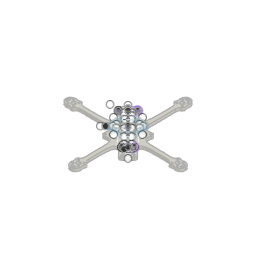
grognatiny (Autodesk Fusion 360 design; units mm, degrees)
Autodesk Fusion 360 part; units mm, degrees
(part 1 of 2)
sketch "Sketch1" plane through (0, 0, 0) normal (0, 0, 1) x (1, 0, 0)
  circle A0 centre (55.82676, 0) radius 4.5 construction
  line L0 (0, 0) -> (55.82676, 0) construction
  line L1 (55.82676, 0) -> (52.64478, 3.181981) construction
  line L2 (219.66262, 222.035886) -> (219.66262, 222.035886)
  circle A1 centre (52.64478, 3.181981) radius 1.05
  circle A2 centre (55.82676, 0) radius 2.25
  line L3 (45.82676, 2) -> (45.82676, -2) construction
  line L4 (55.82676, 0) -> (61.381639, 0) construction
  spline S0 degree 5 poles (60.950506, 0) (60.950506, -0.153969) (60.950156, -0.460974) (60.948561, -0.918704) (60.952621, -1.510726) (61.007799, -2.153667) (61.155369, -2.62162) (61.412622, -2.857725) (61.767904, -2.839751) (62.117367, -2.642136) (62.39542, -2.343591) (62.593133, -1.996472) (62.724237, -1.640351) (62.815846, -1.297091) (62.886296, -0.972425) (62.940492, -0.658247) (62.96936, -0.404167) (62.980649, -0.205879) (62.983159, -0.06935) (62.983159, 0) knots 0 0 0 0 0 0 0.06666667 0.13333333 0.2 0.26666667 0.33333333 0.4 0.46666667 0.53333333 0.6 0.66666667 0.73333333 0.8 0.86666667 0.93333333 1 1 1 1 1 1
  line L5 (60.950506, 0.838643) -> (60.950506, -0.838643)
  line L6 (62.983159, -0.583098) -> (62.983159, 0.583098)
  line L7 (61.359965, -2.867913) -> (62.011175, -2.759378)
  spline S1 degree 5 poles (64.574603, 0) (64.572644, 0.038801) (64.562798, 0.142773) (64.530239, 0.377838) (64.452884, 0.828758) (64.306543, 1.51126) (64.114889, 2.188994) (63.874436, 2.76909) (63.568116, 3.236452) (63.173129, 3.625851) (62.669811, 3.989468) (62.049306, 4.369166) (61.323954, 4.759661) (60.524167, 5.116928) (59.690329, 5.382955) (58.866346, 5.505904) (58.092712, 5.460286) (57.399408, 5.271895) (56.799919, 5.026628) (56.288212, 4.829363) (55.83591, 4.771599) (55.387421, 4.896088) (54.85969, 5.161143) (54.173662, 5.470626) (53.317513, 5.703417) (52.338088, 5.746259) (51.50301, 5.517184) (50.992422, 5.015979) (50.690733, 4.314856) (50.363934, 3.527577) (49.689121, 2.787201) (48.614753, 2.333746) (47.394546, 2.114981) (46.382461, 2.028442) (45.82676, 2) knots 0 0 0 0 0 0 0.03333333 0.06666667 0.1 0.13333333 0.16666667 0.2 0.23333333 0.26666667 0.3 0.33333333 0.36666667 0.4 0.43333333 0.46666667 0.5 0.53333333 0.56666667 0.6 0.63333333 0.66666667 0.7 0.73333333 0.76666667 0.8 0.83333333 0.86666667 0.9 0.93333333 0.96666667 1 1 1 1 1 1
  line L8 (54.534529, 5.88764) -> (50.283948, 5.477622)
  line L9 (64.614563, -0.791723) -> (64.534643, 0.791723)
  line L10 (51.4519, 2.287912) -> (40.20162, 1.712088)
  line L11 (0, 0) -> (70.710678, 70.710678) construction
  line L12 (0, 0) -> (88.663621, 0) construction
  line L13 (-12.75, 12.75) -> (12.75, 12.75) construction
  line L14 (12.75, 12.75) -> (12.75, -12.75) construction
  line L15 (12.75, -12.75) -> (-12.75, -12.75) construction
  line L16 (-12.75, -12.75) -> (-12.75, 12.75) construction
  line L17 (12.75, -12.75) -> (-12.75, 12.75) construction
  circle A3 centre (12.75, 12.75) radius 1.05
  circle A4 centre (12.75, -12.75) radius 1.05
  line L18 (12.75, -12.75) -> (20.528175, -20.528175) construction
  line L19 (17.811227, -7.21301) -> (25.827284, -15.229067)
  line L20 (12.75, 12.75) -> (14.789194, 11.799108) construction
  line L21 (12.75, 12.75) -> (15, 12.75) construction
  circle A5 centre (-12.75, 12.75) radius 1.05
  spline S2 degree 5 poles (60.950506, 0) (60.950506, 0.153969) (60.950156, 0.460974) (60.948561, 0.918704) (60.952621, 1.510726) (61.007799, 2.153667) (61.155369, 2.62162) (61.412622, 2.857725) (61.767904, 2.839751) (62.117367, 2.642136) (62.39542, 2.343591) (62.593133, 1.996472) (62.724237, 1.640351) (62.815846, 1.297091) (62.886296, 0.972425) (62.940492, 0.658247) (62.96936, 0.404167) (62.980649, 0.205879) (62.983159, 0.06935) (62.983159, 0) knots 0 0 0 0 0 0 0.06666667 0.13333333 0.2 0.26666667 0.33333333 0.4 0.46666667 0.53333333 0.6 0.66666667 0.73333333 0.8 0.86666667 0.93333333 1 1 1 1 1 1
  line L22 (60.950506, -0.838643) -> (60.950506, 0.838643)
  line L23 (61.359965, 2.867913) -> (62.011175, 2.759378)
  line L24 (62.983159, 0.583098) -> (62.983159, -0.583098)
  circle A6 centre (52.64478, -3.181981) radius 1.05
  circle A7 centre (59.008741, -3.181981) radius 1.05
  circle A8 centre (59.008741, 3.181981) radius 1.05
  spline S3 degree 5 poles (64.574603, 0) (64.572644, -0.038801) (64.562798, -0.142773) (64.530239, -0.377838) (64.452884, -0.828758) (64.306543, -1.51126) (64.114889, -2.188994) (63.874436, -2.76909) (63.568116, -3.236452) (63.173129, -3.625851) (62.669811, -3.989468) (62.049306, -4.369166) (61.323954, -4.759661) (60.524167, -5.116928) (59.690329, -5.382955) (58.866346, -5.505904) (58.092712, -5.460286) (57.399408, -5.271895) (56.799919, -5.026628) (56.288212, -4.829363) (55.83591, -4.771599) (55.387421, -4.896088) (54.85969, -5.161143) (54.173662, -5.470626) (53.317513, -5.703417) (52.338088, -5.746259) (51.50301, -5.517184) (50.992422, -5.015979) (50.690733, -4.314856) (50.363934, -3.527577) (49.689121, -2.787201) (48.614753, -2.333746) (47.394546, -2.114981) (46.382461, -2.028442) (45.82676, -2) knots 0 0 0 0 0 0 0.03333333 0.06666667 0.1 0.13333333 0.16666667 0.2 0.23333333 0.26666667 0.3 0.33333333 0.36666667 0.4 0.43333333 0.46666667 0.5 0.53333333 0.56666667 0.6 0.63333333 0.66666667 0.7 0.73333333 0.76666667 0.8 0.83333333 0.86666667 0.9 0.93333333 0.96666667 1 1 1 1 1 1
  line L25 (64.614563, 0.791723) -> (64.534643, -0.791723)
  line L26 (54.534529, -5.88764) -> (50.283948, -5.477622)
  line L27 (51.4519, -2.287912) -> (40.20162, -1.712088)
  circle A9 centre (24.059516, -16.996833) radius 1
  circle A10 centre (-12.75, 12.75) radius 1.05
  circle A11 centre (-12.75, 12.75) radius 1.05
  circle A12 centre (16.996833, -24.059516) radius 1
  circle A13 centre (12.75, -12.75) radius 1.05
  line L28 (7.21301, -17.811227) -> (15.229067, -25.827284)
  line L29 (-12.75, 12.75) -> (-14.87132, 14.87132) construction
  line L30 (-20.351398, 9.391243) -> (-9.391243, 20.351398) construction
  circle A14 centre (-9.391243, 20.351398) radius 1.05
  circle A15 centre (-20.351398, 9.391243) radius 1.05
  line L31 (-19.113961, 29.013456) -> (-29.013456, 19.113961)
  line L32 (-12.75, 12.75) -> (-38.01289, 38.01289) construction
  line L33 (-19.113961, 29.013456) -> (-17.121572, 29.187767)
  line L34 (-17.121572, 29.187767) -> (-11.250518, 23.316714)
  spline S4 degree 5 poles (-11.250518, 23.316714) (-11.211276, 23.277472) (-11.101631, 23.209721) (-10.843765, 23.140256) (-10.344886, 23.099857) (-9.591497, 23.084425) (-8.987203, 23.055662) (-8.579926, 23.002689) (-8.335917, 22.949769) (-8.220798, 22.918903) knots 0 0 0 0 0 0 0.2 0.4 0.6 0.8 1 1 1 1 1 1
  line L35 (-11.503755, 23.569951) -> (-10.99728, 23.063476)
  arc A16 (11.158957, 11.159053) -> (11.159053, 11.158957) centre (12.749996, 12.750003) ccw
  arc A17 (14.789185, 11.79911) -> (11.799108, 14.789194) centre (12.749996, 12.750003) ccw
  arc A18 (-11.158952, -11.159057) -> (-11.15905, -11.158959) centre (-12.75, -12.75) ccw
  spline S5 degree 5 poles (14.494771, -2.10759) (14.343355, -1.9605) (13.93616, -1.740481) (12.916067, -1.576004) (10.445932, -1.376362) (6.886656, -1.314026) (4.375107, -1.648566) (4.269226, -2.671161) (6.061066, -4.24007) (7.975171, -5.888004) (9.75136, -7.434183) (11.332926, -8.68999) (12.883508, -9.430311) (14.3705, -9.336735) (15.02046, -7.719066) (15.077807, -5.267015) (14.925488, -3.454947) (14.844657, -2.623021) (14.646188, -2.25468) (14.494771, -2.10759) knots 0 0 0 0 0 0 0.06666667 0.13333333 0.2 0.26666667 0.33333333 0.4 0.46666667 0.53333333 0.6 0.66666667 0.73333333 0.8 0.86666667 0.93333333 1 1 1 1 1 1
  line L36 (15.385704, -2.973067) -> (13.603839, -1.242113)
  line L37 (12.070463, -9.536581) -> (15.14078, -8.923192)
  line L38 (3.905406, -1.674852) -> (5.790919, -4.284775)
  spline S6 degree 5 poles (45.82676, 2) (44.613205, 2.055704) (42.231717, 2.154397) (38.796373, 2.264305) (34.48792, 2.340655) (29.564962, 2.364704) (25.140077, 2.394553) (21.292326, 2.545839) (18.136555, 2.973969) (15.858229, 3.892383) (14.634044, 5.55345) (14.365326, 7.577093) (14.472588, 9.52023) (14.663686, 11.007491) (14.789194, 11.799108) knots 0 0 0 0 0 0 0.1 0.2 0.3 0.4 0.5 0.6 0.7 0.8 0.9 1 1 1 1 1 1
  line L39 (19.464763, 2.656725) -> (15.620145, 4.029888)
  spline S7 degree 5 poles (45.82676, -2) (44.827193, -1.979331) (42.838035, -1.94058) (39.884234, -1.890212) (36.026212, -1.844398) (31.461403, -1.857961) (27.322243, -1.990433) (23.791212, -2.294488) (21.031494, -2.818029) (19.143536, -3.592144) (18.111488, -4.616211) (17.803523, -5.592462) (17.75272, -6.383803) (17.781316, -6.933002) (17.811227, -7.21301) knots 0 0 0 0 0 0 0.1 0.2 0.3 0.4 0.5 0.6 0.7 0.8 0.9 1 1 1 1 1 1
  line L40 (49.229252, -2.070355) -> (42.424269, -1.929645)
  circle A19 centre (3.181981, 64.314952) radius 0.877818
  spline S8 degree 5 poles (0, 69.880814) (-0.038791, 69.878856) (-0.142727, 69.869014) (-0.377693, 69.83647) (-0.828417, 69.759153) (-1.510678, 69.612883) (-2.188281, 69.421327) (-2.768378, 69.18101) (-3.235783, 68.874892) (-3.625179, 68.480187) (-3.988685, 67.977235) (-4.368185, 67.357152) (-4.758537, 66.63222) (-5.115834, 65.8328) (-5.382156, 64.999231) (-5.505663, 64.175387) (-5.460771, 63.401752) (-5.272974, 62.708326) (-5.027875, 62.10863) (-4.830207, 61.596709) (-4.771489, 61.144287) (-4.894829, 60.69597) (-5.159088, 60.168849) (-5.468546, 59.483837) (-5.702258, 58.628791) (-5.746853, 57.65023) (-5.519566, 56.814537) (-5.019245, 56.30421) (-4.318009, 56.003969) (-3.529822, 55.679948) (-2.788231, 55.008781) (-2.333994, 53.93758) (-2.114957, 52.719645) (-2.028407, 51.708998) (-2, 51.153996) knots 0 0 0 0 0 0 0.03333333 0.06666667 0.1 0.13333333 0.16666667 0.2 0.23333333 0.26666667 0.3 0.33333333 0.36666667 0.4 0.43333333 0.46666667 0.5 0.53333333 0.56666667 0.6 0.63333333 0.66666667 0.7 0.73333333 0.76666667 0.8 0.83333333 0.86666667 0.9 0.93333333 0.96666667 1 1 1 1 1 1
  line L41 (0.791723, 69.920774) -> (-0.791723, 69.840854)
  line L42 (-5.88764, 59.84074) -> (-5.477622, 55.590159)
  line L43 (-2.287912, 56.779136) -> (-1.712088, 45.528856)
  circle A20 centre (-3.181981, 57.950991) radius 1.05
  spline S9 degree 5 poles (0, 66.256717) (-0.153969, 66.256717) (-0.460974, 66.256368) (-0.918704, 66.254772) (-1.510726, 66.258832) (-2.153667, 66.314011) (-2.62162, 66.461581) (-2.857725, 66.718834) (-2.839751, 67.074116) (-2.642136, 67.423578) (-2.343591, 67.701631) (-1.996472, 67.899344) (-1.640351, 68.030448) (-1.297091, 68.122057) (-0.972425, 68.192508) (-0.658247, 68.246703) (-0.404167, 68.275572) (-0.205879, 68.286861) (-0.06935, 68.28937) (0, 68.28937) knots 0 0 0 0 0 0 0.06666667 0.13333333 0.2 0.26666667 0.33333333 0.4 0.46666667 0.53333333 0.6 0.66666667 0.73333333 0.8 0.86666667 0.93333333 1 1 1 1 1 1
  line L44 (0.838643, 66.256717) -> (-0.838643, 66.256717)
  line L45 (-2.867913, 66.666176) -> (-2.759378, 67.317386)
  line L46 (-0.583098, 68.28937) -> (0.583098, 68.28937)
  line L47 (2, 51.111947) -> (-2, 51.153996) construction
  spline S10 degree 5 poles (0, 69.880814) (0.038812, 69.878855) (0.14282, 69.869004) (0.377983, 69.83643) (0.829099, 69.759038) (1.511842, 69.612625) (2.189706, 69.420875) (2.769801, 69.180285) (3.237121, 68.873763) (3.626523, 68.478493) (3.990251, 67.97481) (4.370147, 67.353883) (4.760785, 66.628111) (5.11802, 65.827957) (5.383751, 64.993851) (5.506141, 64.169729) (5.459799, 63.396096) (5.270815, 62.702916) (5.025382, 62.103633) (4.828524, 61.59214) (4.771715, 61.139959) (4.897353, 60.691296) (5.163199, 60.162954) (5.4727, 59.475907) (5.704566, 58.618652) (5.745652, 57.638368) (5.514796, 56.803902) (5.012716, 56.293046) (4.31171, 55.989908) (3.52534, 55.660334) (2.786176, 54.981882) (2.3335, 53.904349) (2.115004, 52.68187) (2.028478, 51.668347) (2, 51.111947) knots 0 0 0 0 0 0 0.03333333 0.06666667 0.1 0.13333333 0.16666667 0.2 0.23333333 0.26666667 0.3 0.33333333 0.36666667 0.4 0.43333333 0.46666667 0.5 0.53333333 0.56666667 0.6 0.63333333 0.66666667 0.7 0.73333333 0.76666667 0.8 0.83333333 0.86666667 0.9 0.93333333 0.96666667 1 1 1 1 1 1
  line L48 (-0.791723, 69.920774) -> (0.791723, 69.840854)
  line L49 (5.88764, 59.84074) -> (5.477622, 55.590159)
  line L50 (2.287912, 56.737087) -> (1.712088, 45.486807)
  spline S11 degree 5 poles (-2, 51.153996) (-1.976331, 48.832179) (-1.940518, 44.492019) (-1.921376, 38.89215) (-1.96704, 33.161796) (-2.156464, 28.437921) (-2.498076, 25.588451) (-3.013738, 24.036051) (-3.721992, 23.262032) (-4.629004, 22.869298) (-5.719721, 22.629002) (-6.693811, 22.575138) (-7.451042, 22.679063) (-7.963023, 22.826002) (-8.220798, 22.918903) knots 0 0 0 0 0 0 0.1 0.2 0.3 0.4 0.5 0.6 0.7 0.8 0.9 1 1 1 1 1 1
  line L51 (17.530639, -4.586321) -> (18.091816, -9.8397)
  line L52 (-2.071855, 57.209277) -> (-1.917815, 42.098829)
  line L53 (-5.528897, 21.895138) -> (-10.948173, 23.848226)
  circle A21 centre (-3.181981, 64.314952) radius 1.05
  circle A22 centre (3.181981, 57.950991) radius 1.05
  spline S12 degree 5 poles (0, 66.256717) (0.153969, 66.256717) (0.460974, 66.256368) (0.918704, 66.254772) (1.510726, 66.258832) (2.153667, 66.314011) (2.62162, 66.461581) (2.857725, 66.718834) (2.839751, 67.074116) (2.642136, 67.423578) (2.343591, 67.701631) (1.996472, 67.899344) (1.640351, 68.030448) (1.297091, 68.122057) (0.972425, 68.192508) (0.658247, 68.246703) (0.404167, 68.275572) (0.205879, 68.286861) (0.06935, 68.28937) (0, 68.28937) knots 0 0 0 0 0 0 0.06666667 0.13333333 0.2 0.26666667 0.33333333 0.4 0.46666667 0.53333333 0.6 0.66666667 0.73333333 0.8 0.86666667 0.93333333 1 1 1 1 1 1
  line L54 (-0.838643, 66.256717) -> (0.838643, 66.256717)
  line L55 (2.867913, 66.666176) -> (2.759378, 67.317386)
  line L56 (0.583098, 68.28937) -> (-0.583098, 68.28937)
  spline S13 degree 5 poles (2, 51.111947) (2.068188, 48.352136) (2.184566, 43.289511) (2.299144, 37.066375) (2.343847, 31.281527) (2.295288, 27.021822) (2.254581, 24.3132) (2.364344, 21.885278) (2.792719, 19.044691) (3.727477, 15.925215) (5.367948, 14.340532) (7.402549, 14.201611) (9.406313, 14.429935) (10.964458, 14.656861) (11.799108, 14.789192) knots 0 0 0 0 0 0 0.1 0.2 0.3 0.4 0.5 0.6 0.7 0.8 0.9 1 1 1 1 1 1
  line L57 (50.089428, 1.804339) -> (41.564093, 2.195661)
  line L58 (14.013441, 6.906205) -> (15.564947, 16.692011)
  line L59 (1.804339, 58.02772) -> (2.220188, 41.196821)
  line L60 (2.656725, 19.464763) -> (4.029888, 15.620145)
  line L61 (6.906205, 14.013439) -> (16.692012, 15.564945)
  line L62 (-9.037019, 23.13775) -> (-7.404577, 22.700057)
  spline S14 degree 5 poles (-2.112095, 4.144017) (-1.954309, 4.052667) (-1.697428, 3.995763) (-1.467075, 4.331517) (-1.329791, 5.713841) (-1.300306, 8.600881) (-1.303387, 11.998965) (-1.323089, 15.137048) (-1.416122, 17.416622) (-1.686273, 18.48793) (-2.359754, 18.77531) (-3.528769, 18.782217) (-5.057151, 18.588904) (-6.729113, 18.210793) (-8.292702, 17.603627) (-9.570703, 16.864036) (-10.450454, 16.148134) (-10.885229, 15.55621) (-10.788753, 14.914902) (-10.191069, 13.817591) (-9.714061, 12.754763) (-9.862385, 12.224718) (-9.722625, 11.653536) (-8.672873, 10.507519) (-6.897977, 8.816319) (-4.837238, 6.812143) (-3.402716, 5.340273) (-2.644145, 4.543863) (-2.269882, 4.235367) (-2.112095, 4.144017) knots 0 0 0 0 0 0 0.04 0.08 0.12 0.16 0.2 0.24 0.28 0.32 0.36 0.4 0.44 0.48 0.52 0.56 0.6 0.64 0.68 0.72 0.76 0.8 0.84 0.88 0.92 0.96 1 1 1 1 1 1
  line L63 (-2.632445, 4.445272) -> (-1.591746, 3.842762)
  line L64 (-10.821164, 16.715274) -> (-10.738988, 13.8854)
  line L65 (-1.204223, 17.311809) -> (-2.299533, 19.16541)
  spline S15 degree 5 poles (2, -45.82676) (1.979331, -44.827193) (1.94058, -42.838035) (1.890212, -39.884234) (1.844398, -36.026212) (1.857961, -31.461403) (1.990433, -27.322243) (2.294488, -23.791212) (2.818029, -21.031494) (3.592144, -19.143536) (4.616211, -18.111488) (5.592462, -17.803523) (6.383803, -17.75272) (6.933002, -17.781316) (7.21301, -17.811227) knots 0 0 0 0 0 0 0.1 0.2 0.3 0.4 0.5 0.6 0.7 0.8 0.9 1 1 1 1 1 1
  line L66 (2.070355, -49.229252) -> (1.929645, -42.424269)
  line L67 (4.586321, -17.530639) -> (9.8397, -18.091816)
  spline S16 degree 5 poles (-2, -45.82676) (-2.055704, -44.613205) (-2.154397, -42.231717) (-2.264305, -38.796373) (-2.340655, -34.48792) (-2.364704, -29.564962) (-2.394553, -25.140077) (-2.545839, -21.292326) (-2.973969, -18.136555) (-3.892383, -15.858229) (-5.55345, -14.634044) (-7.577093, -14.365326) (-9.52023, -14.472588) (-11.007491, -14.663686) (-11.799108, -14.789194) knots 0 0 0 0 0 0 0.1 0.2 0.3 0.4 0.5 0.6 0.7 0.8 0.9 1 1 1 1 1 1
  line L68 (-1.804339, -50.089428) -> (-2.195661, -41.564093)
  line L69 (-2.656725, -19.464763) -> (-4.029888, -15.620145)
  line L70 (-6.906205, -14.013441) -> (-16.692011, -15.564947)
  arc A23 (-14.789194, -11.799108) -> (-11.79911, -14.789185) centre (-12.750003, -12.749996) ccw
  circle A24 centre (-12.75, -12.75) radius 1.05
  spline S17 degree 5 poles (0, -64.574603) (-0.038801, -64.572644) (-0.142773, -64.562798) (-0.377838, -64.530239) (-0.828758, -64.452884) (-1.51126, -64.306543) (-2.188994, -64.114889) (-2.76909, -63.874436) (-3.236452, -63.568116) (-3.625851, -63.173129) (-3.989468, -62.669811) (-4.369166, -62.049306) (-4.759661, -61.323954) (-5.116928, -60.524167) (-5.382955, -59.690329) (-5.505904, -58.866346) (-5.460286, -58.092712) (-5.271895, -57.399408) (-5.026628, -56.799919) (-4.829363, -56.288212) (-4.771599, -55.83591) (-4.896088, -55.387421) (-5.161143, -54.85969) (-5.470626, -54.173662) (-5.703417, -53.317513) (-5.746259, -52.338088) (-5.517184, -51.50301) (-5.015979, -50.992422) (-4.314856, -50.690733) (-3.527577, -50.363934) (-2.787201, -49.689121) (-2.333746, -48.614753) (-2.114981, -47.394546) (-2.028442, -46.382461) (-2, -45.82676) knots 0 0 0 0 0 0 0.03333333 0.06666667 0.1 0.13333333 0.16666667 0.2 0.23333333 0.26666667 0.3 0.33333333 0.36666667 0.4 0.43333333 0.46666667 0.5 0.53333333 0.56666667 0.6 0.63333333 0.66666667 0.7 0.73333333 0.76666667 0.8 0.83333333 0.86666667 0.9 0.93333333 0.96666667 1 1 1 1 1 1
  line L71 (0.791723, -64.614563) -> (-0.791723, -64.534643)
  line L72 (-5.88764, -54.534529) -> (-5.477622, -50.283948)
  line L73 (-2.287912, -51.4519) -> (-1.712088, -40.20162)
  spline S18 degree 5 poles (0, -64.574603) (0.038801, -64.572644) (0.142773, -64.562798) (0.377838, -64.530239) (0.828758, -64.452884) (1.51126, -64.306543) (2.188994, -64.114889) (2.76909, -63.874436) (3.236452, -63.568116) (3.625851, -63.173129) (3.989468, -62.669811) (4.369166, -62.049306) (4.759661, -61.323954) (5.116928, -60.524167) (5.382955, -59.690329) (5.505904, -58.866346) (5.460286, -58.092712) (5.271895, -57.399408) (5.026628, -56.799919) (4.829363, -56.288212) (4.771599, -55.83591) (4.896088, -55.387421) (5.161143, -54.85969) (5.470626, -54.173662) (5.703417, -53.317513) (5.746259, -52.338088) (5.517184, -51.50301) (5.015979, -50.992422) (4.314856, -50.690733) (3.527577, -50.363934) (2.787201, -49.689121) (2.333746, -48.614753) (2.114981, -47.394546) (2.028442, -46.382461) (2, -45.82676) knots 0 0 0 0 0 0 0.03333333 0.06666667 0.1 0.13333333 0.16666667 0.2 0.23333333 0.26666667 0.3 0.33333333 0.36666667 0.4 0.43333333 0.46666667 0.5 0.53333333 0.56666667 0.6 0.63333333 0.66666667 0.7 0.73333333 0.76666667 0.8 0.83333333 0.86666667 0.9 0.93333333 0.96666667 1 1 1 1 1 1
  line L74 (-0.791723, -64.614563) -> (0.791723, -64.534643)
  line L75 (5.88764, -54.534529) -> (5.477622, -50.283948)
  line L76 (2.287912, -51.4519) -> (1.712088, -40.20162)
  circle A25 centre (3.181981, -52.64478) radius 1.05
  circle A26 centre (-3.181981, -52.64478) radius 1.05
  circle A27 centre (-3.181981, -59.008741) radius 1.05
  spline S19 degree 5 poles (0, -60.950506) (0.153969, -60.950506) (0.460974, -60.950156) (0.918704, -60.948561) (1.510726, -60.952621) (2.153667, -61.007799) (2.62162, -61.155369) (2.857725, -61.412622) (2.839751, -61.767904) (2.642136, -62.117367) (2.343591, -62.39542) (1.996472, -62.593133) (1.640351, -62.724237) (1.297091, -62.815846) (0.972425, -62.886296) (0.658247, -62.940492) (0.404167, -62.96936) (0.205879, -62.980649) (0.06935, -62.983159) (0, -62.983159) knots 0 0 0 0 0 0 0.06666667 0.13333333 0.2 0.26666667 0.33333333 0.4 0.46666667 0.53333333 0.6 0.66666667 0.73333333 0.8 0.86666667 0.93333333 1 1 1 1 1 1
  line L77 (-0.838643, -60.950506) -> (0.838643, -60.950506)
  line L78 (2.867913, -61.359965) -> (2.759378, -62.011175)
  line L79 (0.583098, -62.983159) -> (-0.583098, -62.983159)
  spline S20 degree 5 poles (0, -60.950506) (-0.153969, -60.950506) (-0.460974, -60.950156) (-0.918704, -60.948561) (-1.510726, -60.952621) (-2.153667, -61.007799) (-2.62162, -61.155369) (-2.857725, -61.412622) (-2.839751, -61.767904) (-2.642136, -62.117367) (-2.343591, -62.39542) (-1.996472, -62.593133) (-1.640351, -62.724237) (-1.297091, -62.815846) (-0.972425, -62.886296) (-0.658247, -62.940492) (-0.404167, -62.96936) (-0.205879, -62.980649) (-0.06935, -62.983159) (0, -62.983159) knots 0 0 0 0 0 0 0.06666667 0.13333333 0.2 0.26666667 0.33333333 0.4 0.46666667 0.53333333 0.6 0.66666667 0.73333333 0.8 0.86666667 0.93333333 1 1 1 1 1 1
  line L80 (0.838643, -60.950506) -> (-0.838643, -60.950506)
  line L81 (-2.867913, -61.359965) -> (-2.759378, -62.011175)
  line L82 (-0.583098, -62.983159) -> (0.583098, -62.983159)
  circle A28 centre (0, -55.82676) radius 2.25
  circle A29 centre (3.181981, -59.008741) radius 1.05
  line L83 (-29.187767, 17.121572) -> (-23.316714, 11.250518)
  spline S21 degree 5 poles (-23.316714, 11.250518) (-23.277472, 11.211276) (-23.209721, 11.101631) (-23.140256, 10.843765) (-23.099857, 10.344886) (-23.084425, 9.591497) (-23.055662, 8.987203) (-23.002689, 8.579926) (-22.949769, 8.335917) (-22.918903, 8.220798) knots 0 0 0 0 0 0 0.2 0.4 0.6 0.8 1 1 1 1 1 1
  line L84 (-23.569951, 11.503755) -> (-23.063476, 10.99728)
  line L85 (-23.13775, 9.037019) -> (-22.700057, 7.404577)
  line L86 (-29.013456, 19.113961) -> (-29.187767, 17.121572)
  spline S22 degree 5 poles (2.10759, -14.494771) (1.9605, -14.343355) (1.740481, -13.93616) (1.576004, -12.916067) (1.376362, -10.445932) (1.314026, -6.886656) (1.648566, -4.375107) (2.671161, -4.269226) (4.24007, -6.061066) (5.888004, -7.975171) (7.434183, -9.75136) (8.68999, -11.332926) (9.430311, -12.883508) (9.336735, -14.3705) (7.719066, -15.02046) (5.267015, -15.077807) (3.454947, -14.925488) (2.623021, -14.844657) (2.25468, -14.646188) (2.10759, -14.494771) knots 0 0 0 0 0 0 0.06666667 0.13333333 0.2 0.26666667 0.33333333 0.4 0.46666667 0.53333333 0.6 0.66666667 0.73333333 0.8 0.86666667 0.93333333 1 1 1 1 1 1
  line L87 (2.973067, -15.385704) -> (1.242113, -13.603839)
  line L88 (1.674852, -3.905406) -> (4.284775, -5.790919)
  line L89 (9.536581, -12.070463) -> (8.923192, -15.14078)
  line L90 (24.059516, -16.996833) -> (16.996833, -24.059516) construction
  line L91 (-9.83936, 13.197667) -> (-9.763065, 11.481026)
  spline S23 degree 5 poles (-4.144017, 2.112095) (-4.052667, 1.954309) (-3.995763, 1.697428) (-4.331517, 1.467075) (-5.713841, 1.329791) (-8.600881, 1.300306) (-11.998965, 1.303387) (-15.137048, 1.323089) (-17.416622, 1.416122) (-18.48793, 1.686273) (-18.77531, 2.359754) (-18.782217, 3.528769) (-18.588904, 5.057151) (-18.210793, 6.729113) (-17.603627, 8.292702) (-16.864036, 9.570703) (-16.148134, 10.450454) (-15.55621, 10.885229) (-14.914902, 10.788753) (-13.817591, 10.191069) (-12.754763, 9.714061) (-12.224718, 9.862385) (-11.653536, 9.722625) (-10.507519, 8.672873) (-8.816319, 6.897977) (-6.812143, 4.837238) (-5.340273, 3.402716) (-4.543863, 2.644145) (-4.235367, 2.269882) (-4.144017, 2.112095) knots 0 0 0 0 0 0 0.04 0.08 0.12 0.16 0.2 0.24 0.28 0.32 0.36 0.4 0.44 0.48 0.52 0.56 0.6 0.64 0.68 0.72 0.76 0.8 0.84 0.88 0.92 0.96 1 1 1 1 1 1
  line L92 (-4.445272, 2.632445) -> (-3.842762, 1.591746)
  line L93 (-17.311809, 1.204223) -> (-19.16541, 2.299533)
  line L94 (-16.715274, 10.821164) -> (-13.8854, 10.738988)
  line L95 (-13.197667, 9.83936) -> (-11.481026, 9.763065)
  line L96 (18.776416, -25.815387) -> (25.78622, -18.804731)
  arc A30 (15.229067, -25.827284) -> (18.776416, -25.815387) centre (16.996833, -24.059516) ccw
  arc A31 (18.7646, -22.291749) -> (18.821533, -22.350578) centre (16.996833, -24.059516) ccw construction
  arc A32 (22.350578, -18.821533) -> (22.291749, -18.7646) centre (24.059516, -16.996833) ccw construction
  arc A33 (25.78622, -18.804731) -> (25.827284, -15.229067) centre (24.059516, -16.996833) ccw
  line L97 (-21.755989, 15.052218) -> (-22.466225, 20.55479)
  line L98 (-24.165105, 21.133885) -> (-26.561273, 18.737717)
  line L99 (-26.561273, 17.323504) -> (-23.454868, 14.2171)
  arc A34 (-23.454868, 14.2171) -> (-21.755989, 15.052218) centre (-22.747761, 14.924206) ccw
  arc A35 (-22.466225, 20.55479) -> (-24.165105, 21.133885) centre (-23.457998, 20.426778) ccw
  arc A36 (-26.561273, 18.737717) -> (-26.561273, 17.323504) centre (-25.854166, 18.030611) ccw
  line L100 (-21.133885, 24.165105) -> (-18.737717, 26.561273)
  arc A37 (-17.323504, 26.561273) -> (-18.737717, 26.561273) centre (-18.030611, 25.854166) ccw
  line L101 (-17.323504, 26.561273) -> (-14.2171, 23.454868)
  arc A38 (-15.052218, 21.755989) -> (-14.2171, 23.454868) centre (-14.924206, 22.747761) ccw
  line L102 (-15.052218, 21.755989) -> (-20.55479, 22.466225)
  arc A39 (-21.133885, 24.165105) -> (-20.55479, 22.466225) centre (-20.426778, 23.457998) ccw
  line L103 (-18.940836, 17.799074) -> (-18.301876, 13.689472)
  line L104 (-16.606642, 13.135999) -> (-14.87132, 14.87132)
  arc A40 (-18.301876, 13.689472) -> (-16.606642, 13.135999) centre (-17.313749, 13.843106) ccw
  line L105 (-17.799074, 18.940836) -> (-13.689472, 18.301876)
  line L106 (-13.135999, 16.606642) -> (-14.87132, 14.87132)
  arc A41 (-13.135999, 16.606642) -> (-13.689472, 18.301876) centre (-13.843106, 17.313749) ccw
  arc A42 (-17.799074, 18.940836) -> (-18.940836, 17.799074) centre (-17.952708, 17.952708) ccw
  line L107 (3.616024, 12.016024) -> (8.016024, 12.016024)
  line L108 (12.016024, 8.016024) -> (12.016024, 3.616024)
  line L109 (10.416024, 2.016024) -> (3.616024, 2.016024)
  line L110 (2.016024, 3.616024) -> (2.016024, 10.416024)
  line L111 (2.016024, 12.016024) -> (12.016024, 2.016024) construction
  arc A43 (12.016024, 8.016024) -> (8.016024, 12.016024) centre (8.016024, 8.016024) ccw
  arc A44 (10.416024, 2.016024) -> (12.016024, 3.616024) centre (10.416024, 3.616024) ccw
  arc A45 (2.016024, 3.616024) -> (3.616024, 2.016024) centre (3.616024, 3.616024) ccw
  arc A46 (3.616024, 12.016024) -> (2.016024, 10.416024) centre (3.616024, 10.416024) ccw
  arc A47 (-2.016024, -3.616024) -> (-3.616024, -2.016024) centre (-3.616024, -3.616024) ccw
  line L112 (-3.616024, -2.016024) -> (-10.416024, -2.016024)
  arc A48 (-10.416024, -2.016024) -> (-12.016024, -3.616024) centre (-10.416024, -3.616024) ccw
  line L113 (-12.016024, -3.616024) -> (-12.016024, -8.016024)
  arc A49 (-12.016024, -8.016024) -> (-8.016024, -12.016024) centre (-8.016024, -8.016024) ccw
  line L114 (-8.016024, -12.016024) -> (-3.616024, -12.016024)
  arc A50 (-3.616024, -12.016024) -> (-2.016024, -10.416024) centre (-3.616024, -10.416024) ccw
  line L115 (-2.016024, -10.416024) -> (-2.016024, -3.616024)
  line L116 (20.528175, -20.528175) -> (19.666109, -21.390492)
  line L117 (18.7646, -22.291749) -> (18.764839, -22.291989)
  line L118 (13.103813, -16.639347) -> (14.871321, -14.871321)
  line L119 (14.286344, -21.40862) -> (12.441612, -19.56458)
  line L120 (15.225673, -22.296741) -> (15.196578, -22.325841)
  line L121 (12.441311, -17.301716) -> (14.871321, -14.871321)
  line L122 (22.320945, -15.200344) -> (22.262752, -15.258547)
  arc A51 (12.441311, -17.301716) -> (12.441612, -19.56458) centre (13.572771, -18.432998) ccw
  arc A52 (17.934791, -21.742615) -> (16.034138, -21.753438) centre (16.997632, -24.060315) ccw
  arc A53 (14.286344, -21.40862) -> (16.034138, -21.753438) centre (15.417502, -20.277037) ccw
  arc A54 (17.934791, -21.742615) -> (19.666109, -21.390492) centre (18.534573, -20.259287) ccw
  line L123 (16.639347, -13.103813) -> (14.871321, -14.871321)
  line L124 (17.301716, -12.441311) -> (14.871321, -14.871321)
  arc A55 (19.56458, -12.441612) -> (17.301716, -12.441311) centre (18.432998, -13.572771) ccw
  line L125 (21.40862, -14.286344) -> (19.56458, -12.441612)
  arc A56 (21.753438, -16.034138) -> (21.40862, -14.286344) centre (20.277037, -15.417502) ccw
  arc A57 (21.753438, -16.034138) -> (21.742615, -17.934791) centre (24.060315, -16.997632) ccw
  arc A58 (21.390492, -19.666109) -> (21.742615, -17.934791) centre (20.259287, -18.534573) ccw
  line L126 (20.528175, -20.528175) -> (21.390492, -19.666109)
  line L127 (-3.181981, 64.314952) -> (3.181981, 57.950991) construction
  circle A59 centre (0, 61.132971) radius 2.25
  line L128 (-51.111947, -2) -> (-51.153996, 2) construction
  circle A60 centre (-57.950991, 3.181981) radius 1.05
  spline S24 degree 5 poles (-66.256717, 0) (-66.256717, -0.153969) (-66.256368, -0.460974) (-66.254772, -0.918704) (-66.258832, -1.510726) (-66.314011, -2.153667) (-66.461581, -2.62162) (-66.718834, -2.857725) (-67.074116, -2.839751) (-67.423578, -2.642136) (-67.701631, -2.343591) (-67.899344, -1.996472) (-68.030448, -1.640351) (-68.122057, -1.297091) (-68.192508, -0.972425) (-68.246703, -0.658247) (-68.275572, -0.404167) (-68.286861, -0.205879) (-68.28937, -0.06935) (-68.28937, 0) knots 0 0 0 0 0 0 0.06666667 0.13333333 0.2 0.26666667 0.33333333 0.4 0.46666667 0.53333333 0.6 0.66666667 0.73333333 0.8 0.86666667 0.93333333 1 1 1 1 1 1
  line L129 (-66.256717, 0.838643) -> (-66.256717, -0.838643)
  line L130 (-66.666176, -2.867913) -> (-67.317386, -2.759378)
  line L131 (-68.28937, -0.583098) -> (-68.28937, 0.583098)
  circle A61 centre (-64.314952, 3.181981) radius 1.05
  spline S25 degree 5 poles (-69.880814, 0) (-69.878856, 0.038791) (-69.869014, 0.142727) (-69.83647, 0.377693) (-69.759153, 0.828417) (-69.612883, 1.510678) (-69.421327, 2.188281) (-69.18101, 2.768378) (-68.874892, 3.235783) (-68.480187, 3.625179) (-67.977235, 3.988685) (-67.357152, 4.368185) (-66.63222, 4.758537) (-65.8328, 5.115834) (-64.999231, 5.382156) (-64.175387, 5.505663) (-63.401752, 5.460771) (-62.708326, 5.272974) (-62.10863, 5.027875) (-61.596709, 4.830207) (-61.144287, 4.771489) (-60.69597, 4.894829) (-60.168849, 5.159088) (-59.483837, 5.468546) (-58.628791, 5.702258) (-57.65023, 5.746853) (-56.814537, 5.519566) (-56.30421, 5.019245) (-56.003969, 4.318009) (-55.679948, 3.529822) (-55.008781, 2.788231) (-53.93758, 2.333994) (-52.719645, 2.114957) (-51.708998, 2.028407) (-51.153996, 2) knots 0 0 0 0 0 0 0.03333333 0.06666667 0.1 0.13333333 0.16666667 0.2 0.23333333 0.26666667 0.3 0.33333333 0.36666667 0.4 0.43333333 0.46666667 0.5 0.53333333 0.56666667 0.6 0.63333333 0.66666667 0.7 0.73333333 0.76666667 0.8 0.83333333 0.86666667 0.9 0.93333333 0.96666667 1 1 1 1 1 1
  line L132 (-69.920774, -0.791723) -> (-69.840854, 0.791723)
  line L133 (-59.84074, 5.88764) -> (-55.590159, 5.477622)
  line L134 (-56.779136, 2.287912) -> (-45.528856, 1.712088)
  spline S26 degree 5 poles (-69.880814, 0) (-69.878855, -0.038812) (-69.869004, -0.14282) (-69.83643, -0.377983) (-69.759038, -0.829099) (-69.612625, -1.511842) (-69.420875, -2.189706) (-69.180285, -2.769801) (-68.873763, -3.237121) (-68.478493, -3.626523) (-67.97481, -3.990251) (-67.353883, -4.370147) (-66.628111, -4.760785) (-65.827957, -5.11802) (-64.993851, -5.383751) (-64.169729, -5.506141) (-63.396096, -5.459799) (-62.702916, -5.270815) (-62.103633, -5.025382) (-61.59214, -4.828524) (-61.139959, -4.771715) (-60.691296, -4.897353) (-60.162954, -5.163199) (-59.475907, -5.4727) (-58.618652, -5.704566) (-57.638368, -5.745652) (-56.803902, -5.514796) (-56.293046, -5.012716) (-55.989908, -4.31171) (-55.660334, -3.52534) (-54.981882, -2.786176) (-53.904349, -2.3335) (-52.68187, -2.115004) (-51.668347, -2.028478) (-51.111947, -2) knots 0 0 0 0 0 0 0.03333333 0.06666667 0.1 0.13333333 0.16666667 0.2 0.23333333 0.26666667 0.3 0.33333333 0.36666667 0.4 0.43333333 0.46666667 0.5 0.53333333 0.56666667 0.6 0.63333333 0.66666667 0.7 0.73333333 0.76666667 0.8 0.83333333 0.86666667 0.9 0.93333333 0.96666667 1 1 1 1 1 1
  line L135 (-69.920774, 0.791723) -> (-69.840854, -0.791723)
  line L136 (-59.84074, -5.88764) -> (-55.590159, -5.477622)
  line L137 (-56.737087, -2.287912) -> (-45.486807, -1.712088)
  circle A62 centre (-61.132971, 0) radius 2.25
  circle A63 centre (-57.950991, -3.181981) radius 1.05
  line L138 (-64.314952, 3.181981) -> (-57.950991, -3.181981) construction
  circle A64 centre (-64.314952, -3.181981) radius 0.877818
  spline S27 degree 5 poles (-66.256717, 0) (-66.256717, 0.153969) (-66.256368, 0.460974) (-66.254772, 0.918704) (-66.258832, 1.510726) (-66.314011, 2.153667) (-66.461581, 2.62162) (-66.718834, 2.857725) (-67.074116, 2.839751) (-67.423578, 2.642136) (-67.701631, 2.343591) (-67.899344, 1.996472) (-68.030448, 1.640351) (-68.122057, 1.297091) (-68.192508, 0.972425) (-68.246703, 0.658247) (-68.275572, 0.404167) (-68.286861, 0.205879) (-68.28937, 0.06935) (-68.28937, 0) knots 0 0 0 0 0 0 0.06666667 0.13333333 0.2 0.26666667 0.33333333 0.4 0.46666667 0.53333333 0.6 0.66666667 0.73333333 0.8 0.86666667 0.93333333 1 1 1 1 1 1
  line L139 (-66.256717, -0.838643) -> (-66.256717, 0.838643)
  line L140 (-66.666176, 2.867913) -> (-67.317386, 2.759378)
  line L141 (-68.28937, 0.583098) -> (-68.28937, -0.583098)
  spline S28 degree 5 poles (-51.111947, -2) (-48.352136, -2.068188) (-43.289511, -2.184566) (-37.066375, -2.299144) (-31.281527, -2.343847) (-27.021822, -2.295288) (-24.3132, -2.254581) (-21.885278, -2.364344) (-19.044691, -2.792719) (-15.925215, -3.727477) (-14.340532, -5.367948) (-14.201611, -7.402549) (-14.429935, -9.406313) (-14.656861, -10.964458) (-14.789192, -11.799108) knots 0 0 0 0 0 0 0.1 0.2 0.3 0.4 0.5 0.6 0.7 0.8 0.9 1 1 1 1 1 1
  line L142 (-58.02772, -1.804339) -> (-41.196821, -2.220188)
  line L143 (-19.464763, -2.656725) -> (-15.620145, -4.029888)
  line L144 (-14.013439, -6.906205) -> (-15.564945, -16.692012)
  spline S29 degree 5 poles (-51.153996, 2) (-48.832179, 1.976331) (-44.492019, 1.940518) (-38.89215, 1.921376) (-33.161796, 1.96704) (-28.437921, 2.156464) (-25.588451, 2.498076) (-24.036051, 3.013738) (-23.262032, 3.721992) (-22.869298, 4.629004) (-22.629002, 5.719721) (-22.575138, 6.693811) (-22.679063, 7.451042) (-22.826002, 7.963023) (-22.918903, 8.220798) knots 0 0 0 0 0 0 0.1 0.2 0.3 0.4 0.5 0.6 0.7 0.8 0.9 1 1 1 1 1 1
  line L145 (-57.209277, 2.071855) -> (-42.098829, 1.917815)
  line L146 (-21.895138, 5.528897) -> (-23.848226, 10.948173)
  point P0 (61.68557, -2.813645)
  point P1 (62.766144, -1.47104)
  point P2 (64.092347, 2.194423)
  point P3 (62.476791, 4.099333)
  point P4 (58.305279, 5.449649)
  point P5 (55.827027, 4.817199)
  point P6 (52.409238, 5.682631)
  point P7 (45.82676, 0)
  point P8 (26.038111, -15.439894)
  point P9 (20.528175, -20.528175)
  point P10 (61.68557, 2.813645)
  point P11 (62.766144, 1.47104)
  point P12 (64.092347, -2.194423)
  point P13 (62.476791, -4.099333)
  point P14 (58.305279, -5.449649)
  point P15 (55.827027, -4.817199)
  point P16 (52.409238, -5.682631)
  point P17 (-14.87132, 14.87132)
  point P18 (-24.063708, 24.063708)
  point P19 (4.848163, -2.979813)
  point P20 (13.605622, -9.229887)
  point P21 (17.542454, 3.343306)
  point P22 (19.31183, -3.681431)
  point P23 (-2.194423, 69.398558)
  point P24 (-5.682631, 57.71545)
  point P25 (2.194423, 69.398558)
  point P26 (0, 51.132971)
  point P27 (5.682631, 57.71545)
  point P28 (4.817199, 61.133239)
  point P29 (4.099333, 67.783002)
  point P30 (1.47104, 68.072355)
  point P31 (-2.813645, 66.991781)
  point P32 (-4.099333, 67.783002)
  point P33 (2.813645, 66.991781)
  point P34 (-4.817199, 61.133239)
  point P35 (-5.449649, 63.611491)
  point P36 (-1.47104, 68.072355)
  point P37 (5.449649, 63.611491)
  point P38 (-4.88494, 22.846057)
  point P39 (3.343306, 17.542454)
  point P40 (-1.751878, 18.23861)
  point P41 (-7.290303, 17.958027)
  point P42 (-10.780076, 15.300337)
  point P43 (1.47104, -62.766144)
  point P44 (-1.47104, -62.766144)
  point P45 (3.681431, -19.31183)
  point P46 (-3.343306, -17.542454)
  point P47 (-2.194423, -64.092347)
  point P48 (-4.099333, -62.476791)
  point P49 (-5.449649, -58.305279)
  point P50 (-4.817199, -55.827027)
  point P51 (-5.682631, -52.409238)
  point P52 (2.194423, -64.092347)
  point P53 (4.099333, -62.476791)
  point P54 (5.449649, -58.305279)
  point P55 (4.817199, -55.827027)
  point P56 (5.682631, -52.409238)
  point P57 (2.813645, -61.68557)
  point P58 (-2.813645, -61.68557)
  point P59 (2.979813, -4.848163)
  point P60 (9.229887, -13.605622)
  point P61 (0, 51.132971)
  point P62 (20.528175, -20.528175)
  point P63 (-9.801212, 12.339346)
  point P64 (-18.23861, 1.751878)
  point P65 (-17.958027, 7.290303)
  point P66 (-15.300337, 10.780076)
  point P67 (-12.339346, 9.801212)
  point P68 (12.016024, 12.016024)
  point P69 (7.016024, 7.016024)
  point P70 (-51.132971, 0)
  point P71 (-68.072355, 1.47104)
  point P72 (-51.132971, 0)
  point P73 (-57.71545, 5.682631)
  point P74 (-57.71545, -5.682631)
  point P75 (-69.398558, -2.194423)
  point P76 (-69.398558, 2.194423)
  point P77 (-67.783002, 4.099333)
  point P78 (-63.611491, -5.449649)
  point P79 (-66.991781, -2.813645)
  point P80 (-66.991781, 2.813645)
  point P81 (-61.133239, -4.817199)
  point P82 (-61.133239, 4.817199)
  point P83 (-68.072355, -1.47104)
  point P84 (-63.611491, 5.449649)
  point P85 (-67.783002, -4.099333)
  point P86 (-17.542454, -3.343306)
  point P87 (-22.846057, 4.88494)
  dimension "d1" = 9
  dimension "d13" = 45
  dimension "d16" = 45
  dimension "d19" = 4
  dimension "d20" = 25.5
  dimension "d21" = 25.5
  dimension "d22" = 2.1
  dimension "d24" = 4.5
  dimension "d25" = 2.1
  dimension "d26" = 11
  dimension "d28" = 25
  dimension "d31" = 360
  dimension "d32" = 2.1
  dimension "d34" = 7.5
  dimension "d35" = 2.5
  dimension "d44" = 2
  dimension "d45" = 3
  dimension "d46" = 15.5
  dimension "d47" = 2.1
  dimension "d48" = 2.1
  dimension "d49" = 14
  dimension "d50" = 13
  dimension "d51" = 2
  dimension "d52" = 140
  dimension "d53" = 3.5
  dimension "d76" = 10
  dimension "d79" = 4
  dimension "d80" = 2
  dimension "d81" = 2
  dimension "d82" = 1
  dimension "d83" = 1
  dimension "d84" = 1
  dimension "d85" = 1
  dimension "d86" = 1
  dimension "d119" = 10
  dimension "d120" = 10
  dimension "d121" = 4
  dimension "d122" = 1.6
  dimension "d123" = 1.6
  dimension "d124" = 1.6
  dimension "d126" = 1.6
  dimension "d127" = 2.5
  dimension "d128" = 1.6
  dimension "d129" = 1.6
  dimension "d190" = 4.5
  constraint coincident L0.start L11.start
  constraint coincident L13.end L14.start
  constraint coincident L14.end L15.start
  constraint tangent L19 A32
  constraint parallel L17 L19
  constraint concentric A9 A32
  constraint symmetric L11 A4 A10
  constraint symmetric L17 A4 A13
  constraint symmetric L17 A30 A32
  constraint symmetric L17 A9 A12
  constraint symmetric L17 A10 A11
  constraint coincident L13.start L16.end
  constraint parallel L17 L29
  constraint perpendicular L17 L30
  constraint parallel L30 L31
  constraint parallel L29 L32
  constraint parallel L32 L34
  constraint concentric A16 A17
  constraint parallel L34 L35
  constraint symmetric A1 L17 A26
  constraint symmetric A2 L17 A28
  constraint symmetric L17 A3 A24
  constraint symmetric L17 A6 A25
  constraint symmetric L17 A7 A29
  constraint symmetric L17 A8 A27
  constraint symmetric L17 A17 A23
  constraint perpendicular L18 L90
  constraint concentric A30 A31
  constraint concentric A32 A33
  constraint parallel L31 L98
  constraint parallel L83 L99
  constraint tangent L97 A34
  constraint tangent L99 A34
  constraint tangent L97 A35
  constraint tangent L98 A35
  constraint tangent L98 A36
  constraint tangent L99 A36
  constraint symmetric L32 A34 A38
  constraint symmetric L32 A35 A39
  constraint symmetric L32 A36 A37
  constraint tangent L104 A40
  constraint tangent L103 A40
  constraint symmetric L32 A40 A41
  constraint tangent L105 A42
  constraint tangent L103 A42
  constraint horizontal L107
  constraint vertical L108
  constraint horizontal L109
  constraint vertical L110
  constraint tangent L108 A43
  constraint tangent L107 A43
  constraint tangent L109 A44
  constraint tangent L108 A44
  constraint tangent L109 A45
  constraint tangent L110 A45
  constraint tangent L110 A46
  constraint tangent L107 A46
  constraint symmetric L17 A43 A49
  constraint symmetric L17 A44 A50
  constraint symmetric L17 A45 A47
  constraint symmetric L17 A46 A48
  constraint perpendicular L116 L117
  constraint parallel L116 L118
  constraint parallel L121 L122
  constraint collinear L120 L122
  constraint tangent L121 A51
  constraint tangent L119 A51
  constraint tangent L117 A52
  constraint tangent L120 A52
  constraint tangent A52 A53
  constraint tangent L119 A53
  constraint tangent A52 A54
  constraint tangent L116 A54
  constraint symmetric L18 A51 A55
  constraint symmetric L18 A52 A57
  constraint symmetric L18 A53 A56
  constraint symmetric L18 A54 A58
  constraint symmetric L32 A19 A64
  constraint symmetric L32 A20 A60
  constraint symmetric L32 A21 A61
  constraint symmetric L32 A22 A63
  constraint symmetric L32 A59 A62
  measures "d1" diameter of A0
  measures "d13" angle of L0 L1
  measures "d16" angle of L11 L12
  measures "d20" distance of L13.start L13.end
  measures "d21" distance of L13.start L15.end
  measures "d22" diameter of A3
  measures "d24" diameter of A16
  measures "d25" diameter of A4
  measures "d28" angle of L20 L21
  measures "d32" diameter of A1
  measures "d35" radius of A32
  measures "d44" diameter of A9
  measures "d47" diameter of A14
  measures "d48" diameter of A15
  measures "d52" angle of L31 L33
  measures "d80" distance of L83 L99
  measures "d81" distance of L31 L98
  measures "d82" radius of A34
  measures "d83" radius of A35
  measures "d84" radius of A36
  measures "d85" radius of A40
  measures "d86" radius of A42
  measures "d121" radius of A43
  measures "d122" radius of A44
  measures "d123" radius of A45
  measures "d124" radius of A46
  measures "d126" radius of A51
  measures "d127" radius of A52
  measures "d128" radius of A53
  measures "d129" radius of A54
  measures "d190" diameter of A59
extrude "Extrude1" add sketch "Sketch1" along normal blind 3 contours S1 L19 S3 L28 L31 L33 L34 S4 L35 A16 A18 S6 S7 S8 L43 S10 L50 S11 S13 L59 S15 S16 S17 S18 L83 S21 L84 L86 L96 A30 A33 S25 L134 S26 L137 S28 L142 S29 | A16 A17 L58 | A16 A17 L58 L61 | A16 A17 L61 | L50 S13 L59 | A18 L70 A23 L144 | A18 L70 A23 | A18 A23 L144 | L137 S28 L142 picked at (30.373981, 0.905159) picked at (14.921814, 12.324338) picked at (12.446326, 14.515395) picked at (12.406768, 14.914922) picked at (2.061892, 47.938075) picked at (-12.44632, -14.515397) picked at (-12.510937, -14.924055) picked at (-14.891386, -12.30487) picked at (-47.938075, -2.061892) makes body 1
ref_plane "WorkPlane1" through (-2.653106, 2.653106, 11) normal (0, 0, 1) x (1, 0, 0)